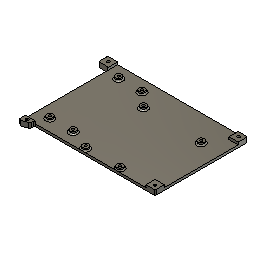
Compact_Robot_MB2 v1 (Autodesk Fusion 360 design; units mm, degrees)
Autodesk Fusion 360 part; units mm, degrees
sketch "Sketch1" plane through (0, 0, 0) normal (0, 1, 0) x (1, 0, 0)
  line L0 (52.75, -37.53) -> (-52.75, -37.53)
  line L1 (-52.75, -37.53) -> (-52.75, 37.53)
  line L2 (-52.75, 37.53) -> (52.75, 37.53)
  line L3 (52.75, 37.53) -> (52.75, -37.53)
  line L4 (52.75, -37.53) -> (-52.75, 37.53) construction
  line L5 (-52.75, -37.53) -> (52.75, 37.53) construction
  dimension "d1" = 105.5
  dimension "d2" = 75.06
  constraint horizontal L0
  constraint perpendicular L0 L1
  constraint parallel L0 L2
  constraint parallel L1 L3
  constraint coincident L4 origin
  constraint coincident L5 origin
  measures "d1" distance of L1.end L2.end
  measures "d2" distance of L0.end L1.end
extrude "Extrude1" add sketch "Sketch1" along normal blind 2
sketch "Sketch2" plane through (0, 2, 0) normal (0, 1, 0) x (-1, 0, 0)
  line L0 (-52.75, -37.53) -> (52.75, -37.53)
  line L1 (52.75, -37.53) -> (52.75, 37.53)
  line L2 (52.75, 37.53) -> (-52.75, 37.53)
  line L3 (-52.75, 37.53) -> (-52.75, -37.53)
  line L4 (52.75, 37.53) -> (52.75, 41.93)
  line L5 (52.75, 41.93) -> (50.89, 43.19)
  line L6 (50.89, 43.19) -> (46.18, 41.3)
  line L7 (46.18, 41.3) -> (45.25, 39.93)
  line L8 (45.25, 39.93) -> (45.25, 38.53)
  line L9 (45.25, 38.53) -> (44.25, 37.53)
  line L10 (52.75, 37.53) -> (44.25, 37.53)
  circle A0 centre (49, 39.88) radius 1.125
  dimension "d5" = 4.4
  dimension "d6" = 1.26
  dimension "d7" = 1.86
  dimension "d8" = 4.71
  dimension "d9" = 1.89
  dimension "d10" = 0.93
  dimension "d11" = 1.37
  dimension "d12" = 1.4
  dimension "d13" = 1
  dimension "d14" = 3.75
  dimension "d15" = 2.25
  dimension "d16" = 2.35
  constraint coincident L1.end L2.start
  constraint perpendicular L2 L4
  constraint vertical L8
  constraint coincident L2 L9.end
  constraint perpendicular L1 L10
  measures "d5" distance of L1.end L4.end
  measures "d6" vertical distance of L4.end L5.end
  measures "d7" horizontal distance of L4.end L5.end
  measures "d8" horizontal distance of L5.end L6.end
  measures "d9" vertical distance of L5.end L6.end
  measures "d10" horizontal distance of L6.end L7.end
  measures "d11" vertical distance of L6.end L7.end
  measures "d12" distance of L7.end L8.end
  measures "d13" horizontal distance of L8.end L9.end
  measures "d14" distance of L4 A0.centre
  measures "d15" diameter of A0
  measures "d16" distance of L10 A0.centre
extrude "Extrude2" add sketch "Sketch2" along normal blind 2 and the other way blind 2 contours L2 L4 L5 L6 L7 L8 L9 L10
sketch "Sketch3" plane through (0, 0, 0) normal (0, -1, 0) x (1, 0, 0)
  circle A0 centre (-49, 39.88) radius 1.125
  line L0 (-52.75, -37.53) -> (52.75, -37.53)
  line L1 (52.75, -37.53) -> (52.75, 37.53)
  line L2 (52.75, 37.53) -> (-44.25, 37.53)
  line L3 (-44.25, 37.53) -> (-45.25, 38.53)
  line L4 (-45.25, 38.53) -> (-45.25, 39.93)
  line L5 (-45.25, 39.93) -> (-46.18, 41.3)
  line L6 (-46.18, 41.3) -> (-50.89, 43.19)
  line L7 (-50.89, 43.19) -> (-52.75, 41.93)
  line L8 (-52.75, 41.93) -> (-52.75, -37.53)
  line L9 (-52.75, -37.53) -> (-60.75, -37.53)
  line L10 (-60.75, -37.53) -> (-60.75, -30.03)
  line L11 (-60.75, -30.03) -> (-52.75, -30.03)
  line L12 (-52.75, -30.03) -> (-52.75, -37.53)
  line L13 (-60.75, -36.53) -> (-59.75, -37.53)
  line L14 (-60.75, -31.03) -> (-59.75, -30.03)
  line L15 (-53.75, -30.03) -> (-52.75, -29.03)
  circle A1 centre (-56.75, -33.78) radius 1.125
  dimension "d21" = 8
  dimension "d22" = 7.5
  dimension "d23" = 8
  dimension "d24" = 7.5
  dimension "d25" = 1
  dimension "d26" = 1
  dimension "d27" = 1
  dimension "d28" = 1
  dimension "d29" = 1
  dimension "d30" = 1
  dimension "d31" = 2.25
  dimension "d32" = 4
  dimension "d33" = 3.75
  constraint coincident L0.start L8.end
  constraint perpendicular L8 L9
  constraint perpendicular L9 L10
  constraint perpendicular L8 L11
  constraint perpendicular L9 L12
  constraint coincident L10 L13.start
  constraint coincident L9 L13.end
  constraint coincident L10 L14.start
  constraint coincident L11 L14.end
  constraint coincident L11 L15.start
  constraint coincident L8 L15.end
  measures "d21" distance of L0.start L9.end
  measures "d22" distance of L9.end L10.end
  measures "d23" distance of L10.end L11.end
  measures "d24" distance of L0.start L11.end
  measures "d25" horizontal distance of L13.start L13.end
  measures "d26" vertical distance of L13.start L13.end
  measures "d27" vertical distance of L14.start L14.end
  measures "d28" horizontal distance of L14.start L14.end
  measures "d29" horizontal distance of L15.start L15.end
  measures "d30" vertical distance of L15.start L15.end
  measures "d31" diameter of A1
  measures "d32" distance of L12 A1.centre
  measures "d33" distance of L9 A1.centre
extrude "Extrude3" add sketch "Sketch3" against normal blind 4 contours L8 L9 L10 L11 L12 L13 L14 | L8 L11 L15
sketch "Sketch4" plane through (0, 0, 0) normal (0, -1, 0) x (1, 0, 0)
  circle A0 centre (-56.75, -33.78) radius 1.125
  circle A1 centre (-49, 39.88) radius 1.125
  line L0 (-59.75, -37.53) -> (52.75, -37.53)
  line L1 (52.75, -37.53) -> (52.75, 37.53)
  line L2 (52.75, 37.53) -> (-44.25, 37.53)
  line L3 (-44.25, 37.53) -> (-45.25, 38.53)
  line L4 (-45.25, 38.53) -> (-45.25, 39.93)
  line L5 (-45.25, 39.93) -> (-46.18, 41.3)
  line L6 (-46.18, 41.3) -> (-50.89, 43.19)
  line L7 (-50.89, 43.19) -> (-52.75, 41.93)
  line L8 (-52.75, 41.93) -> (-52.75, -29.03)
  line L9 (-52.75, -29.03) -> (-53.75, -30.03)
  line L10 (-53.75, -30.03) -> (-59.75, -30.03)
  line L11 (-59.75, -30.03) -> (-60.75, -31.03)
  line L12 (-60.75, -31.03) -> (-60.75, -36.53)
  line L13 (-60.75, -36.53) -> (-59.75, -37.53)
  line L14 (52.75, 37.53) -> (45.25, 37.53)
  line L15 (45.25, 37.53) -> (45.25, 30.03)
  line L16 (45.25, 30.03) -> (52.75, 30.03)
  line L17 (52.75, 30.03) -> (52.75, 37.53)
  line L18 (52, 37.53) -> (52.75, 36.78)
  circle A2 centre (49.25, 34.03) radius 1.125
  line L19 (0, 0) -> (57, 0)
  line L20 (52, -37.53) -> (52.75, -36.78)
  line L21 (45.25, -30.03) -> (52.75, -30.03)
  line L22 (45.25, -37.53) -> (45.25, -30.03)
  line L23 (52.75, -37.53) -> (45.25, -37.53)
  circle A3 centre (49.25, -34.03) radius 1.125
  line L24 (52.75, -30.03) -> (52.75, -37.53)
  point P0 (52.75, -37.53)
  dimension "d36" = 7.5
  dimension "d37" = 7.5
  dimension "d38" = 0.75
  dimension "d39" = 0.75
  dimension "d40" = 4
  dimension "d41" = 4
  dimension "d42" = 2.25
  constraint horizontal L14
  constraint vertical L15
  constraint horizontal L16
  constraint vertical L17
  constraint coincident L1.end L2.start
  constraint coincident L14 L18.start
  constraint coincident L17 L18.end
  constraint coincident L19.start origin
  constraint perpendicular L1 L19
  constraint symmetric L1.end L19 P0
  constraint symmetric L14.end L19 L22.start
  constraint symmetric L15.end L19 L21.start
  constraint symmetric L16.end L19 L21.end
  constraint symmetric L18.start L19 L20.start
  constraint symmetric L18.end L19 L20.end
  constraint symmetric A2 L19 A3
  measures "d36" distance of L1.end L14.end
  measures "d37" distance of L1.end L16.end
  measures "d38" vertical distance of L18.start L18.end
  measures "d39" horizontal distance of L18.start L18.end
  measures "d40" distance of L15 A2.centre
  measures "d41" distance of L16 A2.centre
  measures "d42" diameter of A2
extrude "Extrude4" cut sketch "Sketch4" against normal blind 2 contours L0 L1 L20 L23 L24 | L1 L2 L14 L17 L18
extrude "Extrude5" add sketch "Sketch4" against normal blind 2 from surface at -2 contours L0 L1 L20 L21 L22 L23 L24 | L1 L2 L14 L15 L16 L17 L18
extrude "Extrude6" cut sketch "Sketch4" against normal blind 2 contours A2 | A3
sketch "Sketch5" plane through (0, 0, 0) normal (0, -1, 0) x (1, 0, 0)
  circle A0 centre (49.25, 34.03) radius 1.125
  circle A1 centre (49.25, -34.03) radius 1.125
  line L0 (52.75, 36.78) -> (52, 37.53)
  line L1 (52, 37.53) -> (-44.25, 37.53)
  line L2 (-44.25, 37.53) -> (-45.25, 38.53)
  line L3 (-45.25, 38.53) -> (-45.25, 39.93)
  line L4 (-45.25, 39.93) -> (-46.18, 41.3)
  line L5 (-46.18, 41.3) -> (-50.89, 43.19)
  line L6 (-50.89, 43.19) -> (-52.75, 41.93)
  line L7 (-52.75, 41.93) -> (-52.75, -29.03)
  line L8 (-52.75, -29.03) -> (-53.75, -30.03)
  line L9 (-53.75, -30.03) -> (-59.75, -30.03)
  line L10 (-59.75, -30.03) -> (-60.75, -31.03)
  line L11 (-60.75, -31.03) -> (-60.75, -36.53)
  line L12 (-60.75, -36.53) -> (-59.75, -37.53)
  line L13 (-59.75, -37.53) -> (52, -37.53)
  line L14 (52, -37.53) -> (52.75, -36.78)
  line L15 (52.75, -36.78) -> (52.75, 36.78)
  circle A2 centre (-56.75, -33.78) radius 1.125
  circle A3 centre (-49, 39.88) radius 1.125
  circle A4 centre (-49, 39.88) radius 2
  circle A5 centre (-56.75, -33.78) radius 2
  circle A6 centre (49.25, -34.03) radius 2
  circle A7 centre (49.25, 34.03) radius 2
  dimension "d50" = 4
  dimension "d51" = 4
  dimension "d52" = 4
  dimension "d53" = 4
  constraint concentric A3 A4
  constraint concentric A2 A5
  constraint concentric A1 A6
  constraint concentric A0 A7
  measures "d50" diameter of A4
  measures "d51" diameter of A5
  measures "d52" diameter of A6
  measures "d53" diameter of A7
extrude "Extrude7" cut sketch "Sketch5" against normal blind 3 contours A4 | A5 | A6 | A7
sketch "Sketch6" plane through (0, 2, 0) normal (0, 1, 0) x (-1, 0, 0)
  line L0 (-45.25, 37.53) -> (-45.25, 30.03)
  line L1 (-45.25, 30.03) -> (-52.75, 30.03)
  line L2 (-52.75, 30.03) -> (-52.75, -30.03)
  line L3 (-52.75, -30.03) -> (-45.25, -30.03)
  line L4 (-45.25, -30.03) -> (-45.25, -37.53)
  line L5 (-45.25, -37.53) -> (52.75, -37.53)
  line L6 (52.75, -37.53) -> (52.75, -29.03)
  line L7 (52.75, -29.03) -> (52.75, 37.53)
  line L8 (52.75, 37.53) -> (44.25, 37.53)
  line L9 (44.25, 37.53) -> (-45.25, 37.53)
  circle A0 centre (42.4, 27.94) radius 1
  circle A1 centre (23.4, 27.94) radius 1
  circle A2 centre (6.68, 34.6) radius 1
  circle A3 centre (-21.28, 34.6) radius 1
  circle A4 centre (42.4, 27.94) radius 2.5
  circle A5 centre (23.4, 27.94) radius 2.5
  circle A6 centre (6.68, 34.6) radius 2.5
  circle A7 centre (-21.28, 34.6) radius 2.5
  circle A8 centre (42.4, -27.94) radius 1
  circle A9 centre (23.4, -27.94) radius 1
  circle A10 centre (11.72, -17.46) radius 1
  circle A11 centre (-36.53, -16.18) radius 1
  circle A12 centre (42.4, -27.94) radius 2.5
  circle A13 centre (23.4, -27.94) radius 2.5
  circle A14 centre (11.72, -17.46) radius 2.5
  circle A15 centre (-36.53, -16.18) radius 2.5
  dimension "d56" = 2.93
  dimension "d57" = 2.93
  dimension "d58" = 2
  dimension "d59" = 2
  dimension "d60" = 9.59
  dimension "d61" = 9.59
  dimension "d62" = 2
  dimension "d63" = 2
  dimension "d64" = 10.35
  dimension "d65" = 29.35
  dimension "d66" = 46.07
  dimension "d67" = 74.03
  dimension "d68" = 5
  dimension "d69" = 5
  dimension "d70" = 5
  dimension "d71" = 5
  dimension "d72" = 2
  dimension "d73" = 2
  dimension "d74" = 2
  dimension "d75" = 2
  dimension "d76" = 9.59
  dimension "d77" = 9.59
  dimension "d78" = 20.07
  dimension "d79" = 21.35
  dimension "d80" = 10.35
  dimension "d81" = 29.35
  dimension "d82" = 41.03
  dimension "d83" = 89.28
  dimension "d84" = 5
  dimension "d85" = 5
  dimension "d86" = 5
  dimension "d87" = 5
  constraint concentric A0 A4
  constraint concentric A1 A5
  constraint concentric A2 A6
  constraint concentric A3 A7
  constraint concentric A8 A12
  constraint concentric A9 A13
  constraint concentric A10 A14
  constraint concentric A11 A15
  measures "d56" distance of L9 A2.centre
  measures "d57" distance of L9 A3.centre
  measures "d58" diameter of A3
  measures "d59" diameter of A2
  measures "d60" distance of L9 A1.centre
  measures "d61" distance of L9 A0.centre
  measures "d62" diameter of A1
  measures "d63" diameter of A0
  measures "d64" distance of L7 A0.centre
  measures "d65" distance of L7 A1.centre
  measures "d66" distance of L7 A2.centre
  measures "d67" distance of L7 A3.centre
  measures "d68" diameter of A4
  measures "d69" diameter of A5
  measures "d70" diameter of A6
  measures "d71" diameter of A7
  measures "d72" diameter of A8
  measures "d73" diameter of A9
  measures "d74" diameter of A10
  measures "d75" diameter of A11
  measures "d76" distance of L5 A8.centre
  measures "d77" distance of L5 A9.centre
  measures "d78" distance of L5 A10.centre
  measures "d79" distance of L5 A11.centre
  measures "d80" distance of L7 A8.centre
  measures "d81" distance of L7 A9.centre
  measures "d82" distance of L7 A10.centre
  measures "d83" distance of L7 A11.centre
  measures "d84" diameter of A12
  measures "d85" diameter of A13
  measures "d86" diameter of A14
  measures "d87" diameter of A15
extrude "Extrude8" cut sketch "Sketch6" against normal blind 0.5 contours A0 | A1 | A2 | A3 | A8 | A9 | A10 | A11
extrude "Extrude9" add sketch "Sketch6" along normal blind 2 contours A4 | A5 | A6 | A7 | A12 | A13 | A14 | A15
fillet "Fillet1" radius 1 8 edges at (-40.0692, 2, -27.036) (-21.0692, 2, -27.036) (-9.3892, 2, -16.556) (-40.0692, 2, 28.844) (-21.0692, 2, 28.844) (-4.3492, 2, 35.504) (23.6108, 2, 35.504) (38.8608, 2, -15.276)
